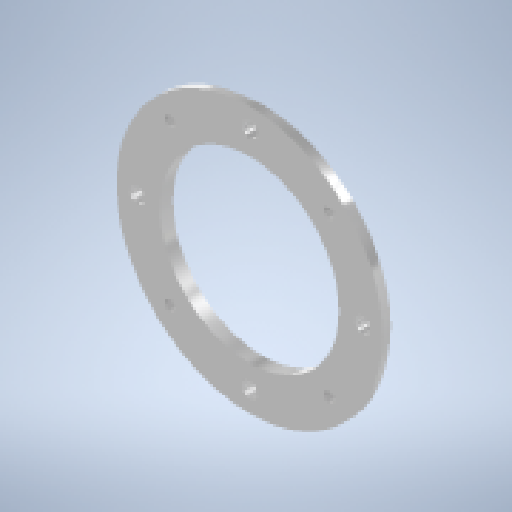
# Autodesk Inventor part: 出力板表
Saved by Autodesk Inventor 2024 (Build 280153000, 153)
## iProperties
Created: 2023-05-29
Part Number: 出力板表
Material: アルミニウム 6061
Document SubType Name: Modeling
Designer: yuta2
Density: 2.7 g/cm^3
Appearance: アルミニウム - フラット
Mass: 56.1952 g
Surface Area: 122.962 cm^2
Volume: 20.8131 cm^3
Author: yuta2
Autodesk Inventor part; units mm, degrees
ref_plane "YZ Plane" through (0, 0, 0) normal (1, 0, 0) x (0, 1, 0)
ref_plane "XZ Plane" through (0, 0, 0) normal (0, 1, 0) x (-1, 0, 0)
ref_plane "XY Plane" through (0, 0, 0) normal (0, 0, 1) x (1, 0, 0)
sketch "スケッチ1" plane through (0, 0, 0) normal (0, 0, 1) x (1, 0, 0)
  circle A0 centre (0, 0) radius 50
  dimension "d0" = 100
  constraints: 1 centre point, 1 coincident
  measures "d0" diameter of A0
extrude "押し出し1" add sketch "スケッチ1" along normal blind 2.5
sketch "スケッチ2" plane through (0, 0, 2.5) normal (0, 0, 1) x (1, 0, 0)
  circle A0 centre (0, 0) radius 52
  dimension "d3" = 104
  constraints: 1 centre point, 1 coincident
  measures "d3" diameter of A0
extrude "押し出し2" add sketch "スケッチ2" along normal blind 2.5
sketch "スケッチ3" plane through (0, 0, 5) normal (0, 0, 1) x (1, 0, 0)
  point P0 (0, 0)
  point P1 (0, 44)
  dimension "d6" = 44
  constraints: 1 vertical alignment
  measures "d6" distance of point (0, 44) point (0, 0)
hole "穴1" at (0, 44, 5) direction (0, 0, -1) diameter 10 end through all
pattern_circular "円形状パターン1" count 4 over 360 about axis through (0, 0, 0) along (0, 0, 1) of "穴1"
sketch "スケッチ4" plane through (0, 0, 5) normal (0, 0, 1) x (1, 0, 0)
  circle A0 centre (0, -44) radius 5 projected
  circle A1 centre (0, 0) radius 44
  line L0 (0, 0) -> (31.1127, 31.1127)
  arc A2 (0, 3.9955) -> (0, 0) centre (1.9978, 1.9978) ccw
  line L1 (0, 3.9955) -> (0, 44)
  dimension "d17" = 45
  constraints: 5 point on circle, 4 end point, 2 centre point, 2 coincident, 2 point on line, 1 vertical
  measures "d17" angle of L1 L0
hole "穴2" at (31.1127, 31.1127, 5) direction (0, 0, -1) diameter 4 end through all
thread "ねじ1" size "M4x0.7" class "6H" standard "ANSI Metric M Profile" full length
pattern_circular "円形状パターン2" count 4 over 360 about axis through (0, 0, 0) along (0, 0, 1) of "穴2"
sketch "スケッチ5" plane through (0, 0, 5) normal (0, 0, 1) x (1, 0, 0)
  circle A0 centre (0, 0) radius 32.5
  dimension "d30" = 65
  constraints: 1 centre point, 1 coincident
  measures "d30" diameter of A0
extrude "押し出し3" cut sketch "スケッチ5" against normal through all
